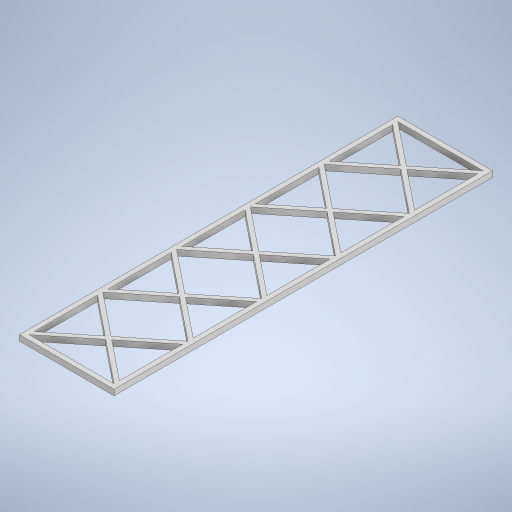
# Autodesk Inventor part: ferris_wheel_main_strut
Saved by Autodesk Inventor 2023 (Build 270158000, 158)
## iProperties
Created: 2025-10-18
Part Number: ferris_wheel_main_strut
Material: Generic
Document SubType Name: Modeling
Designer: Justin Pascual
Density: 1 g/cm^3
Appearance: Default
Author: Justin Pascual
Autodesk Inventor part; units mm, degrees
ref_plane "YZ Plane" through (0, 0, 0) normal (1, 0, 0) x (0, 1, 0)
ref_plane "XZ Plane" through (0, 0, 0) normal (0, 1, 0) x (-1, 0, 0)
ref_plane "XY Plane" through (0, 0, 0) normal (0, 0, 1) x (1, 0, 0)
sketch "Sketch1" plane through (0, 0, 0) normal (0, 1, 0) x (-1, 0, 0)
  line L0 (0, 0) -> (-63.5, 0)
  line L1 (-63.5, 0) -> (-63.5, -254)
  line L2 (-63.5, -254) -> (0, -254)
  line L3 (0, -254) -> (0, 0)
  dimension "d0" = 63.5
  dimension "d1" = 254
  constraints: 8 end point, 2 parallel, 1 horizontal, 1 perpendicular
  measures "d0" distance of L2.end L1.end
  measures "d1" distance of L1.end L0.end
extrude "Extrusion1" add sketch "Sketch1" along normal blind 3.81
sketch "Sketch2" plane through (0, 3.81, 0) normal (0, 1, 0) x (1, 0, 0)
  line L0 (0, 254) -> (0, 0) projected
  line L1 (0, 0) -> (63.5, 0) projected
  line L2 (63.5, 0) -> (63.5, 254) projected
  line L3 (63.5, 254) -> (0, 254) projected
  line L4 (3.175, 3.175) -> (3.175, 250.825)
  line L5 (3.175, 250.825) -> (60.325, 250.825)
  line L6 (60.325, 250.825) -> (60.325, 3.175)
  line L7 (60.325, 3.175) -> (3.175, 3.175)
  line L8 (3.175, 3.175) -> (60.325, 3.175)
  line L9 (60.325, 3.175) -> (60.325, 52.705)
  line L10 (60.325, 52.705) -> (3.175, 52.705)
  line L11 (3.175, 52.705) -> (3.175, 3.175)
  line L12 (3.175, 3.175) -> (3.175, 6.731)
  line L13 (3.175, 6.731) -> (29.5398, 27.94)
  line L14 (60.325, 52.705) -> (60.325, 49.149)
  line L15 (60.325, 49.149) -> (33.9602, 27.94)
  line L16 (3.175, 52.705) -> (3.175, 49.149)
  line L17 (3.175, 49.149) -> (29.5398, 27.94)
  line L18 (60.325, 3.175) -> (60.325, 6.731)
  line L19 (60.325, 6.731) -> (33.9602, 27.94)
  line L20 (31.75, 26.162) -> (3.175, 3.175)
  line L21 (31.75, 29.718) -> (3.175, 52.705)
  line L22 (31.75, 26.162) -> (60.325, 3.175)
  line L23 (31.75, 29.718) -> (60.325, 52.705)
  point P0 (60.325, 3.175)
  dimension "d4" = 3.175
  dimension "d5" = 49.53
  dimension "d6" = 3.556
  dimension "d7" = 3.556
  dimension "d8" = 3.556
  dimension "d9" = 3.556
  constraints: 40 end point, 6 point on line, 2 parallel, 1 horizontal, 1 perpendicular, 3 other
  measures "d4" distance between parallel lines of L0 L4
  measures "d5" distance of L9.end L8.end
  measures "d6" distance of L4.start L12.end
  measures "d7" distance of L9.end L14.end
  measures "d8" distance of L10.end L16.end
  measures "d9" distance of L8.end L18.end
extrude "Extrusion2" cut sketch "Sketch2" against normal blind 6.35 contours L20 L22 L7 | L4 L17 L13 | L19 L15 L6 | L10 L23 L21
pattern_linear "Rectangular Pattern1" count 5 spacing 49.53 along (0, 0, -1) of "Extrusion2"
body "Solid1"
